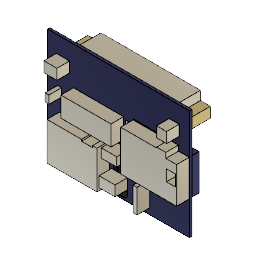
Irrigation unit - PCB board v2 (Autodesk Fusion 360 design; units mm, degrees)
Autodesk Fusion 360 part; units mm, degrees
sketch "Sketch2" plane through (0, 0, 0) normal (0, 1, 0) x (1, 0, 0)
  line L0 (44.704, -13.462) -> (44.704, -21.59)
  line L1 (42.164, -13.462) -> (42.164, -21.59)
  line L2 (49.963, -30.353) -> (49.9687, -30.3243)
  line L3 (52.07, -36.83) -> (52.07, -44.45)
  line L4 (51.689, -31.952) -> (50.038, -31.952)
  line L5 (13.97, -59.182) -> (13.97, -52.578)
  line L6 (49.53, -44.45) -> (49.53, -36.83)
  line L7 (13.97, -52.578) -> (5.588, -52.578)
  line L8 (49.53, -36.83) -> (52.07, -36.83)
  line L9 (42.545, -31.952) -> (42.5163, -31.9463)
  line L10 (49.985, -31.824) -> (50.0093, -31.8077)
  line L11 (51.689, -30.278) -> (51.7177, -30.2837)
  line L12 (7.62, -3.81) -> (7.62, -27.94)
  line L13 (62.23, -19.05) -> (62.23, -13.97)
  line L14 (49.985, -30.406) -> (49.9687, -30.3817)
  line L15 (51.7177, -31.9463) -> (51.689, -31.952)
  line L16 (43.9707, -30.1567) -> (43.995, -30.173)
  line L17 (43.9707, -31.9463) -> (43.942, -31.952)
  line L18 (42.492, -30.173) -> (42.5163, -30.1567)
  line L19 (49.9687, -30.3243) -> (49.985, -30.3)
  line L20 (42.5163, -30.1567) -> (42.545, -30.151)
  line L21 (50.0093, -31.8077) -> (50.038, -31.802)
  line L22 (48.26, -45.72) -> (48.26, -33.02)
  line L23 (43.995, -31.93) -> (43.9707, -31.9463)
  line L24 (8.89, -41.91) -> (6.35, -41.91)
  line L25 (44.0113, -31.9057) -> (43.995, -31.93)
  line L26 (49.9687, -31.8483) -> (49.985, -31.824)
  line L27 (51.742, -31.93) -> (51.7177, -31.9463)
  line L28 (49.963, -31.877) -> (49.9687, -31.8483)
  line L29 (42.545, -31.802) -> (42.545, -30.301)
  line L30 (62.23, -13.97) -> (64.77, -13.97)
  line L31 (50.038, -30.278) -> (51.689, -30.278)
  line L32 (44.017, -31.877) -> (44.0113, -31.9057)
  line L33 (42.5163, -30.2953) -> (42.492, -30.279)
  line L34 (64.77, -13.97) -> (64.77, -19.05)
  line L35 (13.97, -64.77) -> (13.97, -46.99)
  line L36 (49.9687, -30.3817) -> (49.963, -30.353)
  line L37 (44.196, -21.59) -> (42.164, -21.59)
  line L38 (62.23, -13.97) -> (62.23, -8.89)
  line L39 (43.942, -30.151) -> (43.9707, -30.1567)
  line L40 (46.736, -13.462) -> (46.736, -21.59)
  line L41 (42.5163, -31.8077) -> (42.545, -31.802)
  line L42 (51.764, -31.877) -> (51.7583, -31.9057)
  line L43 (8.89, -36.83) -> (8.89, -41.91)
  line L44 (51.7583, -31.9057) -> (51.742, -31.93)
  line L45 (6.35, -41.91) -> (6.35, -36.83)
  line L46 (6.35, -36.83) -> (8.89, -36.83)
  line L47 (44.017, -30.226) -> (44.017, -31.877)
  line L48 (42.492, -31.824) -> (42.5163, -31.8077)
  line L49 (29.53, -29.43) -> (29.53, -31.53)
  line L50 (42.492, -31.93) -> (42.4757, -31.9057)
  line L51 (49.276, -21.59) -> (47.244, -21.59)
  line L52 (50.0093, -30.4223) -> (49.985, -30.406)
  line L53 (42.4757, -30.2547) -> (42.47, -30.226)
  line L54 (49.985, -31.93) -> (49.9687, -31.9057)
  line L55 (40.64, -13.462) -> (40.64, -3.048)
  line L56 (29.53, -28.99) -> (36.51, -28.99)
  line L57 (42.1, -23.84) -> (42.1, -29.49)
  line L58 (29.53, -31.53) -> (36.51, -31.53)
  line L59 (39.37, -27.94) -> (7.62, -27.94)
  line L60 (50.0093, -31.9463) -> (49.985, -31.93)
  line L61 (36.51, -29.43) -> (29.53, -29.43)
  line L62 (42.47, -30.226) -> (42.4757, -30.1973)
  line L63 (36.51, -26.89) -> (29.53, -26.89)
  line L64 (64.77, -3.81) -> (64.77, -8.89)
  line L65 (36.51, -28.99) -> (36.51, -26.89)
  line L66 (42.4757, -30.1973) -> (42.492, -30.173)
  line L67 (36.51, -31.53) -> (36.51, -29.43)
  line L68 (29.53, -26.89) -> (29.53, -28.99)
  line L69 (43.942, -31.952) -> (42.545, -31.952)
  line L70 (44.0113, -30.1973) -> (44.017, -30.226)
  line L71 (48.26, -33.02) -> (16.51, -33.02)
  line L72 (47.244, -13.462) -> (47.244, -21.59)
  line L73 (52.07, -3.81) -> (59.69, -3.81)
  line L74 (0, -69.85) -> (0, 0)
  line L75 (51.7177, -30.2837) -> (51.742, -30.3)
  line L76 (59.69, -3.81) -> (59.69, -11.43)
  line L77 (0, 0) -> (90.17, 0)
  circle A0 centre (45.72, -4.318) radius 1.1359
  line L78 (46.736, -21.59) -> (44.704, -21.59)
  line L79 (90.17, -69.85) -> (0, -69.85)
  line L80 (83.566, -59.182) -> (83.566, -52.578)
  line L81 (39.37, -3.81) -> (7.62, -3.81)
  line L82 (62.23, -8.89) -> (62.23, -3.81)
  line L83 (64.77, -13.97) -> (62.23, -13.97)
  line L84 (77.216, -64.77) -> (13.97, -64.77)
  line L85 (90.17, 0) -> (90.17, -69.85)
  line L86 (62.23, -3.81) -> (64.77, -3.81)
  line L87 (64.77, -8.89) -> (62.23, -8.89)
  line L88 (50.8, -6.858) -> (40.64, -6.858)
  line L89 (83.058, -44.196) -> (83.058, -47.498)
  line L90 (13.97, -46.99) -> (77.216, -46.99)
  line L91 (49.276, -13.462) -> (49.276, -21.59)
  line L92 (44.196, -13.462) -> (44.196, -21.59)
  line L93 (49.022, -1.27) -> (50.8, -3.048)
  line L94 (51.742, -30.3) -> (51.7583, -30.3243)
  line L95 (16.51, -45.72) -> (48.26, -45.72)
  line L96 (77.216, -46.99) -> (77.216, -64.77)
  line L97 (50.8, -3.048) -> (50.8, -13.462)
  line L98 (59.69, -11.43) -> (52.07, -11.43)
  line L99 (83.058, -47.498) -> (54.356, -47.498)
  line L100 (52.07, -11.43) -> (52.07, -3.81)
  line L101 (83.457, -31.5373) -> (83.457, -38.6769)
  line L102 (51.9, -29.49) -> (51.9, -23.84)
  line L103 (77.216, -52.578) -> (83.566, -52.578)
  line L104 (50.038, -31.952) -> (50.0093, -31.9463)
  line L105 (51.9, -23.84) -> (42.1, -23.84)
  line L106 (51.7583, -30.3243) -> (51.764, -30.353)
  line L107 (42.1, -29.49) -> (51.9, -29.49)
  line L108 (62.23, -8.89) -> (64.77, -8.89)
  line L109 (40.64, -3.048) -> (42.418, -1.27)
  line L110 (89.271, -38.6769) -> (89.271, -31.5373)
  line L111 (42.4757, -31.8483) -> (42.492, -31.824)
  line L112 (5.588, -59.182) -> (13.97, -59.182)
  line L113 (54.356, -21.336) -> (89.916, -21.336)
  line L114 (43.995, -30.173) -> (44.0113, -30.1973)
  line L115 (77.216, -52.578) -> (77.216, -59.182)
  line L116 (39.37, -27.94) -> (39.37, -3.81)
  line L117 (49.985, -30.3) -> (50.0093, -30.2837)
  line L118 (42.5163, -31.9463) -> (42.492, -31.93)
  line L119 (16.51, -33.02) -> (16.51, -45.72)
  line L120 (50.8, -13.462) -> (40.64, -13.462)
  line L121 (42.492, -30.279) -> (42.4757, -30.2547)
  line L122 (77.216, -59.182) -> (83.566, -59.182)
  line L123 (50.038, -31.802) -> (50.038, -30.428)
  line L124 (42.545, -30.151) -> (43.942, -30.151)
  line L125 (64.77, -19.05) -> (62.23, -19.05)
  line L126 (49.9687, -31.9057) -> (49.963, -31.877)
  line L127 (83.457, -38.6769) -> (89.271, -38.6769)
  line L128 (52.07, -44.45) -> (49.53, -44.45)
  line L129 (5.588, -52.578) -> (5.588, -59.182)
  line L130 (42.47, -31.877) -> (42.4757, -31.8483)
  line L131 (42.545, -30.301) -> (42.5163, -30.2953)
  line L132 (89.271, -31.5373) -> (83.457, -31.5373)
  line L133 (89.916, -44.196) -> (83.058, -44.196)
  line L134 (50.0093, -30.2837) -> (50.038, -30.278)
  line L135 (42.4757, -31.9057) -> (42.47, -31.877)
  line L136 (54.356, -47.498) -> (54.356, -21.336)
  line L137 (64.77, -8.89) -> (64.77, -13.97)
  line L138 (50.038, -30.428) -> (50.0093, -30.4223)
  line L139 (51.764, -30.353) -> (51.764, -31.877)
  line L140 (89.916, -21.336) -> (89.916, -44.196)
  line L141 (42.418, -1.27) -> (49.022, -1.27)
extrude "Extrude5" add sketch "Sketch2" along normal blind 20 contours L5 L7 L35 L112 L129 | L5 L35 L84 L90 L96 L99 L115 L136 | L80 L96 L103 L115 L122 makes body 1
extrude "Extrude6" add sketch "Sketch2" along normal blind 13 separate body contours L73 L76 L98 L100 makes body 2
extrude "Extrude7" add sketch "Sketch2" along normal blind 6.5 separate body contours L89 L90 L96 L99 L113 L133 L136 L140 | L12 L59 L63 L65 L68 L81 L116 makes body 3 at (25.5067, 0, 11.5033) makes body 4 at (61.976, 0, 38.4387)
extrude "Extrude8" add sketch "Sketch2" along normal blind 15 separate body contours L24 L43 L45 L46 makes body 5
extrude "Extrude9" add sketch "Sketch2" along normal blind 5 separate body contours L0 L40 L78 L120 | L55 L88 L97 L120 | L1 L37 L92 L120 | L51 L72 L91 L120 | L55 L88 L93 L97 L109 L141 | L2 L4 L10 L11 L14 L15 L19 L21 L26 L27 L28 L31 L36 L42 L44 L52 L54 L60 L75 L94 L104 L106 L117 L123 L126 L134 L138 L139 | L3 L6 L8 L128 | L9 L16 L17 L18 L20 L23 L25 L29 L32 L33 L39 L41 L47 L48 L50 L53 L62 L66 L69 L70 L111 L114 L118 L121 L124 L130 L131 L135 | L56 L59 L65 L68 | L13 L30 L34 L83 L125 | L30 L38 L83 L87 L108 L137 | L64 L82 L86 L87 L108 | L22 L71 L95 L119 | L49 L58 L61 L67 | L57 L102 L105 L107 | L101 L110 L127 L132 makes body 6 at (34.1833, 3.3333, 29.43) makes body 7 at (50.5883, 1.6667, 30.278) makes body 8 at (49.4195, 0, 7.156) makes body 9 at (44.017, 1.6667, 30.7763) makes body 10 at (34.1833, 3.3333, 27.94) makes body 11 at (37.6767, 0, 41.4867) makes body 12 at (45.3667, 0, 27.6067) makes body 13 at (62.23, 1.6667, 13.97) makes body 14 at (52.07, 1.6667, 39.37) makes body 15 at (85.395, 0, 33.9172)
extrude "Extrude3" add sketch "Sketch2" along normal blind 1.6 contours L74 L77 L79 L85 bodies 1 2 3 4 5
extrude "Extrude4" add sketch "Sketch2" against normal blind 8 separate body contours L55 L88 L97 L120 | L5 L7 L35 L112 L129 | L89 L90 L96 L99 L113 L133 L136 L140 | L80 L96 L103 L115 L122 | L12 L59 L63 L65 L68 L81 L116 | L13 L30 L34 L83 L125 | L30 L38 L83 L87 L108 L137 | L64 L82 L86 L87 L108 | L22 L71 L95 L119 | L24 L43 L45 L46 | L57 L102 L105 L107 makes body 16 at (62.23, -2.6667, 13.97) makes body 17 at (8.382, -2.6667, 59.182) makes body 18 at (77.216, -5.3333, 54.7793) makes body 19 at (47.4133, -2.6667, 13.462) makes body 20 at (48.6333, -2.6667, 23.84) makes body 21 at (25.5067, 0, 11.5033) makes body 22 at (61.976, 0, 38.4387) makes body 23 at (37.6767, 0, 41.4867) makes body 24 at (6.35, -2.6667, 40.2167)
